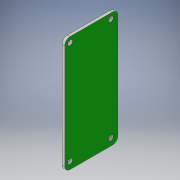
# Autodesk Inventor part: RPI_Zero
Saved by Autodesk Inventor 2018 (Build 220112000, 112)
## iProperties
Created: 2018-09-18
Part Number: RPI_Zero
Material: Generic
Document SubType Name: Modeling
Designer: Viraj Shah
Density: 1 g/cm^3
Appearance: Default
Author: Viraj Shah
Autodesk Inventor part; units mm, degrees
ref_plane "YZ Plane" through (0, 0, 0) normal (1, 0, 0) x (0, 1, 0)
ref_plane "XZ Plane" through (0, 0, 0) normal (0, 1, 0) x (-1, 0, 0)
ref_plane "XY Plane" through (0, 0, 0) normal (0, 0, 1) x (1, 0, 0)
sketch "Sketch1" plane through (0, 0, 0) normal (1, 0, 0) x (0, 1, 0)
  line L0 (-12, 32.5) -> (12, 32.5)
  line L1 (15, 29.5) -> (15, -29.5)
  line L2 (12, -32.5) -> (-12, -32.5)
  line L3 (-15, -29.5) -> (-15, 29.5)
  line L4 (-15, 32.5) -> (15, -32.5) construction
  line L5 (15, 32.5) -> (-15, -32.5) construction
  arc A0 (-12, 32.5) -> (-15, 29.5) centre (-12, 29.5) ccw
  arc A1 (15, 29.5) -> (12, 32.5) centre (12, 29.5) ccw
  arc A2 (12, -32.5) -> (15, -29.5) centre (12, -29.5) ccw
  arc A3 (-15, -29.5) -> (-12, -32.5) centre (-12, -29.5) ccw
  point P0 (0, 0)
  dimension "d0" = 30
  dimension "d1" = 65
  dimension "d22" = 3
  constraints: 12 end point, 8 point on circle, 8 point on line, 8 tangent, 4 centre point, 3 equal radius, 2 midpoint, 2 parallel, 1 horizontal, 1 perpendicular
  measures "d0" distance of L4.end L5.end
  measures "d1" distance of L5.start L4.end
  measures "d22" radius of A0
extrude "Extrusion1" add sketch "Sketch1" along normal blind 1.5
fillet "Fillet1" [suppressed]
sketch "Sketch2" plane through (1.5, 0, 0) normal (1, 0, 0) x (0, 0, -1)
  line L0 (29.5, 15) -> (-29.5, 15) projected
  line L1 (-32.5, 12) -> (-32.5, -12) projected
  arc A0 (-32.5, -12) -> (-29.5, -15) centre (-29.5, -12) ccw projected
  point P0 (0, 0)
  point P1 (-29.5, 11)
  point P2 (32, 15)
  point P3 (-32, 15)
  point P4 (-33, 14)
  point P5 (-33, -14)
  point P6 (28.5, 11)
  point P7 (28.5, -12)
  dimension "d5" = 4
  dimension "d6" = 3
  dimension "d9" = 58
  dimension "d12" = 23
  constraints: 1 horizontal, 1 other
  measures "d5" distance from line of L0 point (-29.5, 11)
  measures "d9" distance of point (-29.5, 11) point (28.5, 11)
  measures "d12" distance of point (-29.5, 11) point (-29.5, -12)
hole "Hole1" at (1.5, 11, 29.5) at (1.5, 11, -28.5) at (1.5, -12, 29.5) at (1.5, -12, -28.5) direction (-1, 0, 0) diameter 2.75 end through all
body "Solid1"
